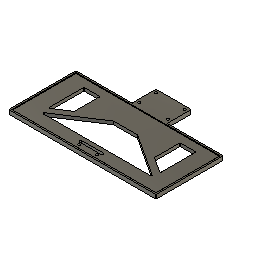
Tracker_solaire_support_celluleR (Autodesk Fusion 360 design; units mm, degrees)
Autodesk Fusion 360 part; units mm, degrees
sketch "Sketch3" plane through (0, 0, 0) normal (0, 0, 1) x (1, 0, 0)
  line L0 (90, 40) -> (-90, 40)
  line L1 (-90, 40) -> (-90, -40)
  line L2 (-90, -40) -> (90, -40)
  line L3 (90, -40) -> (90, 40)
  line L4 (90, 40) -> (-90, -40) construction
  line L5 (-90, 40) -> (90, -40) construction
  line L6 (-92, -42) -> (92, -42)
  line L7 (92, -42) -> (92, 42)
  line L8 (92, 42) -> (-92, 42)
  line L9 (-92, 42) -> (-92, -42)
  dimension "d6" = 180
  dimension "d7" = 80
  dimension "d8" = 2
  constraint horizontal L0
  constraint perpendicular L0 L1
  constraint parallel L0 L2
  constraint parallel L1 L3
  constraint coincident L4 origin
  constraint coincident L5 origin
  measures "d6" distance of L1.end L2.end
  measures "d7" distance of L0.end L1.end
extrude "Extrude2" add sketch "Sketch3" along normal blind 5
extrude "Extrude3" add sketch "Sketch3" along normal blind 4 contours L0 L1 L2 L3
sketch "Sketch6" plane through (0, 0, 5) normal (0, 0, 1) x (-1, 0, 0)
  line L0 (-90, -40) -> (-90, 40)
  line L1 (-90, 40) -> (90, 40)
  line L2 (90, 40) -> (90, -40)
  line L3 (90, -40) -> (-90, -40)
  line L4 (92, -42) -> (92, 42)
  line L5 (92, 42) -> (-92, 42)
  line L6 (-92, 42) -> (-92, -42)
  line L7 (-92, -42) -> (92, -42)
  line L8 (-22, -27) -> (-22, -57)
  line L9 (22, -57) -> (22, -27)
  line L10 (22, -42) -> (-22, -42)
  line L11 (-22, -42) -> (-22, -72)
  line L12 (-22, -72) -> (22, -72)
  line L13 (22, -72) -> (22, -42)
  line L14 (22, -42) -> (-22, -72) construction
  line L15 (-22, -42) -> (22, -72) construction
  point P0 (0, -42)
  point P1 (0, -57)
  dimension "d20" = 44
  dimension "d21" = 30
  dimension "d22" = 44
  dimension "d23" = 30
  constraint parallel L8 L9
  constraint midpoint L7 P0
  constraint horizontal L10
  constraint perpendicular L10 L11
  constraint parallel L10 L12
  constraint parallel L11 L13
  constraint coincident L14 P1
  constraint coincident L15 P1
  measures "d20" distance of L8.end L9.start
  measures "d21" distance of L8.start L8.end
  measures "d22" distance of L11.end L12.end
  measures "d23" distance of L10.end L11.end
extrude "Extrude4" add sketch "Sketch6" against normal blind 5 contours L7 L8 L9 L10 L11 L12 L13
sketch "Sketch7" plane through (0, 0, 5) normal (0, 0, 1) x (-1, 0, 0)
  line L0 (-90, -40) -> (-90, 40)
  line L1 (-90, 40) -> (90, 40)
  line L2 (90, 40) -> (90, -40)
  line L3 (90, -40) -> (-90, -40)
  line L4 (92, -42) -> (92, 42)
  line L5 (92, 42) -> (-92, 42)
  line L6 (-92, 42) -> (-92, -42)
  line L7 (-92, -42) -> (-22, -42)
  line L8 (-22, -42) -> (-22, -72)
  line L9 (-22, -72) -> (22, -72)
  line L10 (22, -72) -> (22, -42)
  line L11 (22, -42) -> (92, -42)
  circle A0 centre (-18, -68) radius 1.5
  circle A1 centre (18, -68) radius 1.5
  circle A2 centre (-18, -47) radius 1.5
  circle A3 centre (18, -47) radius 1.5
  dimension "d26" = 3
  dimension "d27" = 4
  dimension "d28" = 4
  dimension "d29" = 3
  dimension "d30" = 3
  dimension "d31" = 3
  dimension "d32" = 4
  dimension "d33" = 4
  dimension "d34" = 4
  dimension "d35" = 7
  dimension "d36" = 4
  dimension "d37" = 7
  measures "d26" diameter of A0
  measures "d27" distance of L8 A0.centre
  measures "d28" distance of L9 A0.centre
  measures "d29" diameter of A1
  measures "d30" diameter of A2
  measures "d31" diameter of A3
  measures "d32" distance of L10 A1.centre
  measures "d33" distance of L9 A1.centre
  measures "d34" distance of L8 A2.centre
  measures "d35" distance of L3 A2.centre
  measures "d36" distance of L10 A3.centre
  measures "d37" distance of L3 A3.centre
extrude "Extrude5" cut sketch "Sketch7" against normal blind 6 contours A2
extrude "Extrude6" cut sketch "Sketch7" against normal blind 6 contours A0
extrude "Extrude7" cut sketch "Sketch7" against normal blind 23 contours A3
extrude "Extrude8" cut sketch "Sketch7" against normal blind 15 contours A1
sketch "Sketch8" plane through (0, 0, 4) normal (0, 0, 1) x (-1, 0, 0)
  line L0 (-90, 40) -> (-90, -40)
  line L1 (-90, -40) -> (90, -40)
  line L2 (90, -40) -> (90, 40)
  line L3 (90, 40) -> (-90, 40)
  line L4 (15, 29) -> (-15, 29)
  line L5 (-15, 29) -> (-15, 32)
  line L6 (-15, 32) -> (15, 32)
  line L7 (15, 32) -> (15, 29)
  line L8 (15, 29) -> (-15, 32) construction
  line L9 (-15, 29) -> (15, 32) construction
  circle A0 centre (-13.5, 30.5) radius 1.5
  circle A1 centre (13.5, 30.5) radius 1.5
  circle A2 centre (-11, 35) radius 1
  circle A3 centre (11, 35) radius 1
  point P0 (0, 30.5)
  dimension "d46" = 30
  dimension "d47" = 3
  dimension "d48" = 8
  dimension "d49" = 5
  dimension "d50" = 5
  dimension "d51" = 4
  dimension "d52" = 4
  constraint horizontal L4
  constraint perpendicular L4 L5
  constraint parallel L4 L6
  constraint parallel L5 L7
  constraint coincident L8 P0
  constraint coincident L9 P0
  constraint tangent L5 A0
  constraint tangent L4 A0
  constraint tangent L6 A0
  constraint tangent L4 A1
  constraint tangent L7 A1
  constraint tangent L6 A1
  measures "d46" distance of L5.end L6.end
  measures "d47" distance of L4.end L5.end
  measures "d48" distance of L3 L6
  measures "d49" distance of L3 A3.centre
  measures "d50" distance of L3 A2.centre
  measures "d51" distance of L7 A3.centre
  measures "d52" distance of L5 A2.centre
extrude "Extrude9" cut sketch "Sketch8" against normal blind 12 contours L4 L6 A0 A1 | A1 | A0
extrude "Extrude10" cut sketch "Sketch8" against normal blind 25 contours A2 | A3
sketch "Sketch9" plane through (0, 0, 4) normal (0, 0, 1) x (-1, 0, 0)
  circle A0 centre (-11, 35) radius 1
  circle A1 centre (11, 35) radius 1
  line L0 (13.5, 29) -> (-13.5, 29)
  arc A2 (-13.5, 32) -> (-13.5, 29) centre (-13.5, 30.5) ccw
  line L1 (-13.5, 32) -> (13.5, 32)
  arc A3 (13.5, 29) -> (13.5, 32) centre (13.5, 30.5) ccw
  line L2 (-90, 40) -> (-90, -40)
  line L3 (-90, -40) -> (90, -40)
  line L4 (90, -40) -> (90, 40)
  line L5 (90, 40) -> (-90, 40)
  line L6 (70, 24.0265) -> (-70, 24.0265)
  line L7 (0, 24.0265) -> (0, -12)
  line L8 (-70, 24.0265) -> (-15, -12)
  line L9 (15, -12) -> (70, 24.0265)
  line L10 (-15, -12) -> (15, -12)
  line L11 (70, 15) -> (70, -30)
  line L12 (70, -30) -> (50, -30)
  line L13 (70, 15) -> (50, 2)
  line L14 (50, 2) -> (50, -30)
  line L15 (-70, 15) -> (-50, 2)
  line L16 (-70, 15) -> (-70, -30)
  line L17 (-50, 2) -> (-50, -30)
  line L18 (-70, -30) -> (-50, -30)
  point P0 (0, -12)
  dimension "d62" = 28
  constraint horizontal L6
  constraint midpoint L6 L7.start
  constraint coincident P0 L7.end
  constraint horizontal L10
  constraint perpendicular L6 L11
  constraint perpendicular L11 L12
  constraint symmetric L7 L11.start L15.start
  constraint symmetric L7 L11.end L16.end
  constraint symmetric L7 L12.end L17.end
  constraint symmetric L7 L13.end L15.end
  measures "d62" distance of L3 L10
extrude "Extrude11" cut sketch "Sketch9" against normal blind 25 contours L6 L7 L9 L10 | L6 L7 L8 L10
fillet "Fillet1" radius 1 1 edges at (-70, -24.0265, 2)
fillet "Fillet2" radius 1 3 edges at (70, -24.0265, 2) (15, 12, 2) (-15, 12, 2)
extrude "Extrude12" cut sketch "Sketch9" against normal blind 15 contours L11 L12 L13 L14 | L15 L16 L17 L18
fillet "Fillet3" radius 1 4 edges at (70, -15, 2) (50, -2, 2) (50, 30, 2) (70, 30, 2)
fillet "Fillet4" radius 1 4 edges at (-50, -2, 2) (-70, -15, 2) (-70, 30, 2) (-50, 30, 2)
fillet "Fillet5" radius 1 6 edges at (-22, 72, 2.5) (22, 72, 2.5) (-92, 42, 2.5) (-92, -42, 2.5) (92, 42, 2.5) (92, -42, 2.5)
sketch "Sketch11" plane through (0, 0, 4) normal (0, 0, 1) x (-1, 0, 0)
sketch "Sketch12" plane through (0, 0, 4) normal (0, 0, 1) x (-1, 0, 0)
sketch "Sketch13" plane through (0, 0, 4) normal (0, 0, 1) x (-1, 0, 0)
  circle A0 centre (-11, 35) radius 1.5
  circle A1 centre (11, 35) radius 1.5
  dimension "d79" = 3
  dimension "d80" = 3
  measures "d79" diameter of A0
  measures "d80" diameter of A1
extrude "Extrude13" cut sketch "Sketch13" against normal blind 100
